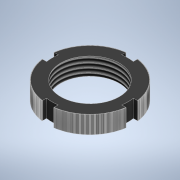
# Autodesk Inventor part: PORCA
Saved by Autodesk Inventor 2022 (Build 260153000, 153)
## iProperties
Created: 2023-07-19
Part Number: PORCA
Material: Generic
Document SubType Name: Modeling
Designer: Usuário
Density: 1 g/cm^3
Appearance: Glossy - Black
Author: Usuário
Autodesk Inventor part; units mm, degrees
ref_plane "YZ Plane" through (0, 0, 0) normal (1, 0, 0) x (0, 1, 0)
ref_plane "XZ Plane" through (0, 0, 0) normal (0, 1, 0) x (-1, 0, 0)
ref_plane "XY Plane" through (0, 0, 0) normal (0, 0, 1) x (1, 0, 0)
sketch "Sketch1" plane through (0, 0, 0) normal (0, 1, 0) x (-1, 0, 0)
  circle A0 centre (0, 0) radius 10
  circle A1 centre (0, 0) radius 14.5
  dimension "d0" = 20
  dimension "d1" = 29
  constraints: 2 centre point, 2 coincident
  measures "d0" diameter of A0
  measures "d1" diameter of A1
extrude "Extrusion1" add sketch "Sketch1" along normal blind 6
sketch "Sketch2" plane through (0, 6, 0) normal (0, 1, 0) x (1, 0, 0)
  line L0 (-16.5843, 0) -> (16.5185, 0) construction
  line L1 (-0.0329, -17.8992) -> (-0.0329, 24.8682) construction
  circle A0 centre (0, 0) radius 14.5 projected
  circle A1 centre (0, 0) radius 13
  line L2 (-14.3614, 2) -> (-12.8452, 2)
  line L3 (-14.3614, -2) -> (-12.8452, -2)
  line L4 (-2.0329, -14.3568) -> (-2.0329, -12.8401)
  line L5 (1.9671, -14.3659) -> (1.9671, -12.8503)
  line L6 (12.8452, -2) -> (14.3614, -2)
  line L7 (12.8452, 2) -> (14.3614, 2)
  line L8 (1.9671, 12.8503) -> (1.9671, 14.3659)
  line L9 (-2.0329, 12.8401) -> (-2.0329, 14.3568)
  dimension "d8" = 1.5
  constraints: 20 end point, 8 parallel, 1 horizontal, 1 vertical, 19 other
sketch "Sketch3" plane through (0, 6, 0) normal (0, 1, 0) x (1, 0, 0)
  arc A0 (1.9671, -14.2145) -> (14.2128, -1.9793) centre (0, 0) ccw
  line L0 (2.0671, -14.2003) -> (2.0671, -14.3528)
  line L1 (1.9671, -14.2145) -> (1.9671, -14.3659)
  line L2 (2.1671, -14.1854) -> (2.1671, -14.3377)
  arc A1 (-14.5, 0) -> (-14.5, 0) centre (0, 0) ccw projected
  circle A2 centre (0, 0) radius 14.5 projected
  line L3 (2.0671, -14.2003) -> (2.1671, -14.1854)
  line L4 (2.0671, -14.3528) -> (2.1671, -14.3377)
  point P0 (2.0671, -14.3519)
  point P1 (2.1671, -14.3371)
  dimension "d13" = 0.1
  dimension "d14" = 0.1
  dimension "d17" = 14.35
  dimension "d19" = 0.15
  constraints: 10 end point, 4 point on circle, 2 point on line, 1 centre point
  measures "d13" distance between parallel lines of L0 L1
  measures "d14" distance between parallel lines of L0 L2
  measures "d17" radius of A0
  measures "d19" radial gap between concentric circles of A1 A0
extrude "Extrusion3" cut sketch "Sketch3" against normal blind 6 contours A0 L2 A1 L0
pattern_circular "Circular Pattern1" count 300 over 360 about axis through (0, 0, 0) along (0, 1, 0) of "Extrusion3"
extrude "Extrusion4" cut sketch "Sketch2" against normal blind 6 contours A0 L6 A1 L7 | L8 A1 L9 A0 | A0 L4 A1 L5 | L2 A1 L3 A0
thread "Thread1" size "M20x1.5" standard "Din Taper" length 8.5
body "Solid1"
